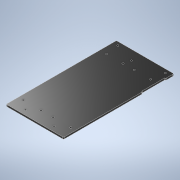
# Autodesk Inventor part: Battery Cover
Saved by Autodesk Inventor 2021 (Build 250183000, 183)
## iProperties
Created: 2020-08-17
Part Number: Battery Cover
Material: Generic
Document SubType Name: Modeling
Designer: jgray
Density: 1 g/cm^3
Appearance: Default
Author: jgray
Autodesk Inventor part; units mm, degrees
ref_plane "YZ Plane" through (0, 0, 0) normal (1, 0, 0) x (0, 1, 0)
ref_plane "XZ Plane" through (0, 0, 0) normal (0, 1, 0) x (-1, 0, 0)
ref_plane "XY Plane" through (0, 0, 0) normal (0, 0, 1) x (1, 0, 0)
sketch "Sketch1" plane through (0, 0, 0) normal (0, 1, 0) x (-1, 0, 0)
  line L0 (0, 0) -> (128.5, 0)
  line L1 (128.5, 0) -> (128.5, -247)
  line L2 (128.5, -247) -> (0, -247)
  line L3 (0, -247) -> (0, 0)
  dimension "d0" = 128.5
  dimension "d1" = 247
  constraints: 8 end point, 2 parallel, 1 horizontal, 1 perpendicular
  measures "d0" distance of L1.end L2.end
  measures "d1" distance of L0.end L1.end
extrude "Extrusion1" add sketch "Sketch1" along normal blind 4
sketch "Sketch2" plane through (0, 4, 0) normal (0, 1, 0) x (1, 0, 0)
  line L0 (0, 0) -> (0, 247) projected
  line L1 (0, 177) -> (-2, 177)
  line L2 (-2, 177) -> (-2, 229)
  line L3 (-2, 229) -> (0, 229)
  line L4 (0, 229) -> (0, 177)
  line L5 (-128.5, 0) -> (0, 0) projected
  line L6 (0, 247) -> (-128.5, 247) projected
  point P0 (0, 229)
  dimension "d6" = 2
  dimension "d9" = 18
  dimension "d10" = 70
  constraints: 8 end point, 2 parallel, 1 horizontal, 1 perpendicular, 1 point on line
  measures "d6" distance between parallel lines of L0 L2
  measures "d9" distance between parallel lines of L6 L3
  measures "d10" distance between parallel lines of L6 L1
extrude "Extrusion2" cut sketch "Sketch2" against normal blind 4
fillet "Fillet1" radius 1 2 edges at (-2, 2, -229) (-2, 2, -177)
sketch "Sketch3" plane through (0, 4, 0) normal (0, 1, 0) x (1, 0, 0)
  line L0 (-117.5, -38.6181) -> (-117.5, 315.6014) construction
  line L1 (-187.6527, 11) -> (40.6594, 11) construction
  line L2 (-11, -30.2243) -> (-11, 315.6014) construction
  line L3 (-64.25, -57.9239) -> (-64.25, 315.6014) construction
  line L4 (-128.5, 0) -> (0, 0) construction
  line L5 (-128.5, 247) -> (-128.5, 0) construction
  line L6 (0, 0) -> (0, 177) construction
  line L7 (-187.6527, 27.25) -> (32.1527, 27.25) construction
  line L8 (0, 247) -> (-128.5, 247) projected
  point P0 (-64.25, 0)
  point P1 (-11, 27.25)
  point P2 (-117.5, 27.25)
  point P3 (-50.75, 27.25)
  point P4 (-77.75, 27.25)
  point P5 (-96.25, 11)
  point P6 (-32.25, 11)
  point P7 (-117.5, 239)
  point P8 (-11, 239)
  point P9 (-72.75, 225)
  dimension "d12" = 11
  dimension "d13" = 11
  dimension "d14" = 11
  dimension "d15" = 27.25
  dimension "d16" = 13.5
  dimension "d17" = 13.5
  dimension "d18" = 32
  dimension "d19" = 32
  dimension "d27" = 8
  dimension "d28" = 8
  dimension "d29" = 8.5
  dimension "d30" = 22
  constraints: 10 end point, 10 point on line, 3 vertical, 2 midpoint, 1 horizontal, 1 perpendicular
  measures "d12" distance between parallel lines of L4 L1
  measures "d13" distance between parallel lines of L5 L0
  measures "d14" distance between parallel lines of L6 L2
  measures "d15" distance between parallel lines of L4 L7
  measures "d16" distance from line of point (-50.75, 27.25) L3
  measures "d17" distance from line of point (-77.75, 27.25) L3
  measures "d18" distance from line of point (-96.25, 11) L3
  measures "d19" distance from line of point (-32.25, 11) L3
  measures "d27" distance from line of L8 point (-117.5, 239)
  measures "d28" distance from line of L8 point (-11, 239)
  measures "d29" distance from line of point (-72.75, 225) L3
  measures "d30" distance from line of L8 point (-72.75, 225)
hole "Hole1" at (-11, 4, -27.25) at (-117.5, 4, -27.25) at (-50.75, 4, -27.25) at (-77.75, 4, -27.25) at (-96.25, 4, -11) at (-32.25, 4, -11) at (-117.5, 4, -239) at (-72.75, 4, -225) at (-11, 4, -239) direction (0, -1, 0) diameter 3.8 end through all
sketch "Sketch4" plane through (0, 4, 0) normal (0, 1, 0) x (1, 0, 0)
  circle A0 centre (-72.75, 225) radius 1.9 projected
  circle A1 centre (-32.25, 11) radius 1.9 projected
  circle A2 centre (-77.75, 27.25) radius 1.9 projected
  circle A3 centre (-117.5, 27.25) radius 1.9 projected
  circle A4 centre (-11, 27.25) radius 1.9 projected
  circle A5 centre (-50.75, 27.25) radius 1.9 projected
  circle A6 centre (-96.25, 11) radius 1.9 projected
  circle A7 centre (-117.5, 239) radius 1.9 projected
  circle A8 centre (-11, 239) radius 1.9 projected
  line L0 (-1, 229) -> (0, 229) projected
  line L1 (0, 229) -> (0, 247) projected
  line L2 (0, 247) -> (-128.5, 247) projected
  line L3 (-128.5, 247) -> (-128.5, 0) projected
  line L4 (-128.5, 0) -> (0, 0) projected
  line L5 (0, 0) -> (0, 177) projected
  line L6 (0, 177) -> (-1, 177) projected
  arc A9 (-2, 178) -> (-1, 177) centre (-1, 178) ccw projected
  line L7 (-2, 178) -> (-2, 228) projected
  arc A10 (-1, 229) -> (-2, 228) centre (-1, 228) ccw projected
  line L8 (-146.6271, 210) -> (41.5181, 210) construction
  line L9 (-64.25, -27.386) -> (-64.25, 314.2803) construction
  point P0 (-64.25, 247)
  point P1 (-113.5, 210)
  point P2 (-76.75, 210)
  point P3 (-51.75, 210)
  point P4 (-15, 210)
  dimension "d31" = 37
  dimension "d32" = 15
  dimension "d33" = 15
  dimension "d34" = 12.5
  dimension "d35" = 12.5
  constraints: 5 point on line, 4 end point, 1 horizontal, 1 midpoint, 1 vertical
  measures "d31" distance between parallel lines of L2 L8
  measures "d32" distance from line of point (-15, 210) L1
  measures "d33" distance from line of L3 point (-113.5, 210)
  measures "d34" distance from line of point (-76.75, 210) L9
  measures "d35" distance from line of point (-51.75, 210) L9
hole "Hole2" at (-113.5, 4, -210) at (-76.75, 4, -210) at (-51.75, 4, -210) at (-15, 4, -210) direction (0, -1, 0) diameter 3.8 end through all
fillet "Fillet2" radius 2 6 edges at (0, 2, -229) (0, 2, -177) (0, 2, -247) (-128.5, 2, -247) (0, 2, 0) (-128.5, 2, 0)
body "Solid1"
